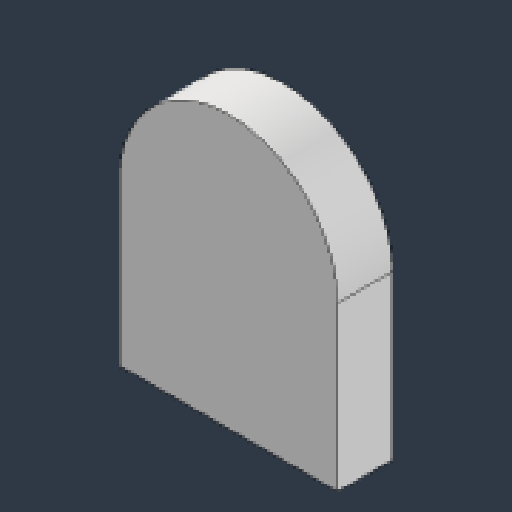
# Autodesk Inventor part: MOUNT,KICKER
Saved by Autodesk Inventor 2026 (Build 300175050, 175E)
## iProperties
Created: 2026-04-12
Part Number: MOUNT,KICKER
Material: Generic
Document SubType Name: Sheet Metal
Designer: Jthib
Mass: 4.68137 g
Surface Area: 21.3103 cm^2
Volume: 4.68137 cm^3
Density: 1 g/cm^3
Sheet Metal Rule: Default
Appearance: Default
Author: Jthib
Autodesk Inventor part; units mm, degrees
ref_plane "YZ Plane" through (0, 0, 0) normal (1, 0, 0) x (0, 1, 0)
ref_plane "XZ Plane" through (0, 0, 0) normal (0, 1, 0) x (-1, 0, 0)
ref_plane "XY Plane" through (0, 0, 0) normal (0, 0, 1) x (1, 0, 0)
sketch "Sketch1" plane through (0, 0, 0) normal (0, 0, 1) x (1, 0, 0)
  line L0 (-17.78, 0) -> (17.78, 0) construction
  line L1 (-12.7, 0) -> (12.7, 0)
  line L2 (12.7, 0) -> (12.7, 19.05)
  arc A0 (12.7, 19.05) -> (-12.7, 19.05) centre (0, 19.05) ccw
  line L3 (-12.7, 19.05) -> (-12.7, 0)
  point P0 (0, 0)
  dimension "d0" = 25.4
  dimension "d1" = 19.05
  constraints: 6 end point, 2 point on circle, 2 tangent, 1 centre point, 1 collinear, 1 horizontal, 1 midpoint, 1 parallel, 1 perpendicular
  measures "d0" distance between parallel lines of L2 L3
  measures "d1" distance of L1.end L2.end
extrude "Extrusion1" add sketch "Sketch1" along normal mid plane 6.35
equation "\"BendRadius\" = Thickness"
equation "\"BendReliefWidth\" = Thickness"
equation "\"BendReliefDepth\" = 0.5 * Thickness"
equation "\"CornerReliefSize\" = 4 * Thickness"
equation "\"MinimumRemnant\" = 2 * Thickness"
equation "\"TransitionRadius\" = BendRadius"
equation "\"JacobiRadiusSize\" = BendRadius"
equation "\"GapSize\" = Thickness"
equation "\"Thickness\" = 3.048"
body "Solid1"
